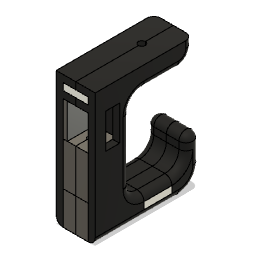
sennheiser_hd280_desk_hanger (Autodesk Fusion 360 design; units mm, degrees)
Autodesk Fusion 360 part; units mm, degrees
note: some values were not read from the file. Set by a fixed rule: which sketch regions a step uses.
sketch "outer_holder" plane through (0, 0, 0) normal (1, 0, 0) x (0, 0, -1)
  line L0 (0, 0) -> (70, 0)
  line L1 (70, 0) -> (70, 0)
  line L2 (60, -10) -> (34.9991, -10)
  line L3 (0, -10) -> (0, 0)
  line L4 (24.9991, -20) -> (24.9991, -65)
  line L5 (24.9991, -90) -> (0, -90)
  line L6 (0, -90) -> (0, -10)
  arc A0 (34.9991, -10) -> (24.9991, -20) centre (34.9991, -20) ccw
  arc A1 (60, -10) -> (70, 0) centre (60, 0) ccw
  line L7 (24.9991, -90) -> (60, -90)
  line L8 (75, -75) -> (75, -75)
  line L9 (55, -75) -> (34.9991, -75)
  line L10 (65, -65) -> (65, -60)
  line L11 (70, -55) -> (70, -55)
  line L12 (75, -60) -> (75, -75)
  arc A2 (70, -55) -> (65, -60) centre (70, -60) ccw
  arc A3 (75, -60) -> (70, -55) centre (70, -60) ccw
  arc A4 (24.9991, -65) -> (34.9991, -75) centre (34.9991, -65) ccw
  arc A5 (55, -75) -> (65, -65) centre (55, -65) ccw
  arc A6 (60, -90) -> (75, -75) centre (60, -75) ccw
  line L13 (7.5, -10) -> (17.5, -10)
  line L14 (17.5, -10) -> (17.5, -35)
  line L15 (17.5, -35) -> (7.5, -35)
  line L16 (7.5, -35) -> (7.5, -10)
  line L17 (35, -85) -> (55, -85)
  line L18 (55, -85) -> (55, -80)
  line L19 (55, -80) -> (35, -80)
  line L20 (35, -80) -> (35, -85)
  line L21 (0, 0) -> (70, 0)
  line L22 (70, 0) -> (70, 5)
  line L23 (70, 5) -> (0, 5)
  line L24 (0, 5) -> (0, 0)
  point P0 (74.9991, -90)
  point P1 (75, -55)
  dimension "d1" = 70
  dimension "d2" = 10
  dimension "d3" = 80
  dimension "d5" = 10
  dimension "d6" = 10
  dimension "d7" = 50
  dimension "d8" = 15
  dimension "d9" = 20
  dimension "d11" = 5
  dimension "d12" = 5
  dimension "d13" = 10
  dimension "d14" = 10
  dimension "d15" = 15
  dimension "d16" = 10
  dimension "d17" = 25
  dimension "d20" = 10
  dimension "d21" = 7.5
  dimension "d55" = 20
  dimension "d56" = 5
  dimension "d122" = 70
  dimension "d123" = 5
  constraint horizontal L0
  constraint horizontal L2
  constraint vertical L3
  constraint coincident L0.start L3.end
  constraint vertical L4
  constraint horizontal L5
  constraint vertical L6
  constraint coincident L3.start L2
  constraint tangent L2 A0
  constraint tangent L4 A0
  constraint tangent L2 A1
  constraint horizontal L7
  constraint horizontal L9
  constraint vertical L10
  constraint vertical L12
  constraint tangent L10 A2
  constraint coincident P1 L12
  constraint coincident P1 L11
  constraint tangent L12 A3
  constraint coincident L5.start L4
  constraint tangent L4 A4
  constraint tangent L9 A4
  constraint coincident L8.start L9
  constraint tangent L10 A5
  constraint tangent L9 A5
  constraint coincident P0 L8
  constraint coincident P0 L7
  constraint tangent L7 A6
  constraint horizontal L13
  constraint vertical L14
  constraint horizontal L15
  constraint vertical L16
  constraint horizontal L17
  constraint vertical L18
  constraint horizontal L19
  constraint vertical L20
  constraint horizontal L21
  constraint vertical L22
  constraint horizontal L23
  constraint vertical L24
  measures "d1" distance of L0.start L0.end
  measures "d2" distance of L0.start L3.start
  measures "d3" distance of L3.start L5.end
  measures "d5" radius of A0
  measures "d6" radius of A1
  measures "d7" distance of L5.start P0
  measures "d8" distance of L7 L9
  measures "d9" distance of L8.start P1
  measures "d11" radius of A2
  measures "d12" radius of A3
  measures "d13" radius of A4
  measures "d14" radius of A5
  measures "d15" radius of A6
  measures "d16" distance of L13.start L13.end
  measures "d17" distance of L13.start L15.end
  measures "d20" distance of L0 L13
  measures "d21" distance of L6 L16
  measures "d55" distance of L17.start L17.end
  measures "d56" distance of L17.start L19.end
  measures "d122" distance of L0.start L0.end
  measures "d123" distance of L0.start L23.end
extrude "Extrude6" add sketch "outer_holder" along normal blind 5 makes body 1
sketch "inner_holder" plane through (5, 0, 0) normal (1, 0, 0) x (0, 0, -1)
  line L0 (15, -35) -> (10, -35)
  line L1 (10, -35) -> (10, -10)
  line L2 (10, -10) -> (15, -10)
  line L3 (15, -10) -> (15, -35)
  line L4 (0, -90) -> (60, -90)
  arc A0 (60, -90) -> (75, -75) centre (60, -75) ccw
  line L5 (75, -75) -> (75, -60)
  arc A1 (75, -60) -> (65, -60) centre (70, -60) ccw
  line L6 (65, -60) -> (65, -65)
  arc A2 (55, -75) -> (65, -65) centre (55, -65) ccw
  line L7 (55, -75) -> (34.9996, -75)
  arc A3 (24.9996, -65) -> (34.9996, -75) centre (34.9996, -65) ccw
  line L8 (24.9996, -65) -> (24.9996, -20)
  arc A4 (34.9996, -10) -> (24.9996, -20) centre (34.9996, -20) ccw
  line L9 (34.9996, -10) -> (60, -10)
  arc A5 (60, -10) -> (70, 0) centre (60, 0) ccw
  line L10 (70, 0) -> (0, 0)
  line L11 (0, 0) -> (0, -55)
  line L12 (0, -55) -> (5, -55)
  line L13 (5, -55) -> (5, -75)
  line L14 (5, -75) -> (0, -75)
  line L15 (0, -75) -> (0, -90)
  line L16 (60, 0) -> (70, 0)
  line L17 (70, 0) -> (70, 0)
  line L18 (0, -10) -> (0, -5)
  arc A6 (60, -10) -> (70, 0) centre (60, 0) ccw
  line L19 (70, -55) -> (70, -55)
  line L20 (65, -60) -> (65, -65)
  line L21 (75, -75) -> (75, -60)
  line L22 (55, -75) -> (35, -75)
  line L23 (20, -90) -> (60, -90)
  line L24 (75, -75) -> (75, -75)
  line L25 (25, -20) -> (25, -65)
  line L26 (20, -90) -> (20, -10)
  arc A7 (35, -10) -> (25, -20) centre (35, -20) ccw
  arc A8 (25, -65) -> (35, -75) centre (35, -65) ccw
  arc A9 (55, -75) -> (65, -65) centre (55, -65) ccw
  arc A10 (70, -55) -> (65, -60) centre (70, -60) ccw
  arc A11 (75, -60) -> (70, -55) centre (70, -60) ccw
  line L27 (0, -10) -> (20, -10)
  arc A12 (60, -90) -> (75, -75) centre (60, -75) ccw
  line L28 (60, 0) -> (60, -10)
  line L29 (35, -10) -> (35, -5)
  line L30 (35, -5) -> (0, -5)
  line L31 (30, -80) -> (60, -80)
  line L32 (60, -80) -> (60, -85)
  line L33 (60, -85) -> (30, -85)
  line L34 (30, -85) -> (30, -80)
  line L35 (17.5, -35) -> (7.5, -35)
  line L36 (7.5, -35) -> (7.5, -10)
  line L37 (7.5, -10) -> (17.5, -10)
  line L38 (17.5, -10) -> (17.5, -35)
  line L39 (35, -85) -> (35, -80)
  line L40 (35, -80) -> (55, -80)
  line L41 (55, -80) -> (55, -85)
  line L42 (55, -85) -> (35, -85)
  line L43 (0, -90) -> (60, -90)
  arc A13 (60, -90) -> (75, -75) centre (60, -75) ccw
  line L44 (75, -75) -> (75, -60)
  arc A14 (75, -60) -> (65, -60) centre (70, -60) ccw
  line L45 (65, -60) -> (65, -65)
  arc A15 (55, -75) -> (65, -65) centre (55, -65) ccw
  line L46 (55, -75) -> (34.9991, -75)
  arc A16 (24.9991, -65) -> (34.9991, -75) centre (34.9991, -65) ccw
  line L47 (24.9991, -65) -> (24.9991, -20)
  arc A17 (34.9991, -10) -> (24.9991, -20) centre (34.9991, -20) ccw
  line L48 (34.9991, -10) -> (60, -10)
  arc A18 (60, -10) -> (70, 0) centre (60, 0) ccw
  line L49 (20, -75) -> (25, -75)
  line L50 (25, -75) -> (25, -85)
  line L51 (25, -85) -> (20, -85)
  line L52 (20, -85) -> (20, -75)
  line L53 (20, -60) -> (25, -60)
  line L54 (25, -60) -> (25, -45)
  line L55 (25, -45) -> (20, -45)
  line L56 (20, -45) -> (20, -60)
  line L57 (70, 0) -> (70, 5)
  line L58 (70, 5) -> (0, 5)
  line L59 (0, 5) -> (0, -90)
  line L60 (60, 0) -> (70, 0)
  line L61 (70, 0) -> (70, 5)
  line L62 (70, 5) -> (60, 5)
  line L63 (60, 5) -> (60, 0)
  dimension "d33" = 10
  dimension "d34" = 10
  dimension "d35" = 10
  dimension "d36" = 10
  dimension "d37" = 5
  dimension "d38" = 5
  dimension "d39" = 15
  dimension "d71" = 5
  dimension "d72" = 10
  dimension "d73" = 5
  dimension "d74" = 15
  dimension "d75" = 5
  dimension "d76" = 35
  dimension "d124" = 10
  dimension "d125" = 5
  constraint horizontal L16
  constraint vertical L18
  constraint vertical L20
  constraint vertical L21
  constraint horizontal L22
  constraint horizontal L23
  constraint coincident L4 L23.start
  constraint vertical L25
  constraint vertical L26
  constraint tangent L25 A7
  constraint tangent L25 A8
  constraint tangent L22 A8
  constraint coincident A0.end L22
  constraint tangent L20 A9
  constraint tangent L22 A9
  constraint tangent L20 A10
  constraint tangent L21 A11
  constraint tangent L23 A12
  constraint coincident A5.centre L16.start
  constraint perpendicular L9 L29
  constraint perpendicular L18 L30
  constraint horizontal L31
  constraint vertical L32
  constraint horizontal L33
  constraint vertical L34
  constraint horizontal L49
  constraint vertical L50
  constraint horizontal L51
  constraint vertical L52
  constraint coincident L26 L49.start
  constraint horizontal L53
  constraint vertical L54
  constraint horizontal L55
  constraint vertical L56
  constraint coincident L26 L53.start
  constraint horizontal L60
  constraint vertical L61
  constraint horizontal L62
  constraint vertical L63
  measures "d33" radius of A6
  measures "d34" radius of A7
  measures "d35" radius of A8
  measures "d36" radius of A9
  measures "d37" radius of A10
  measures "d38" radius of A11
  measures "d39" radius of A12
  measures "d71" distance of L49.start L49.end
  measures "d72" distance of L49.start L51.end
  measures "d73" distance of L23 L51
  measures "d74" distance of L53.start L55.end
  measures "d75" distance of L53.start L53.end
  measures "d76" distance of L9 L55
  measures "d124" distance of A5.centre A5.end
  measures "d125" distance of A5.centre L62.end
extrude "Extrude13" add sketch "inner_holder" along normal blind 9 contours L2 L8 A4 L11 L18 L25 L26 A7 L27 L29 L30 L37 L47 A17 L55 L59 bodies 1
extrude "Extrude14" add sketch "inner_holder" along normal blind 9 contours L4 A0 L5 A1 L6 A2 L7 A3 L8 L20 L21 L22 L23 L25 L26 A8 A9 A10 A11 A12 L43 A13 L44 A14 L45 A15 L46 A16 L47 L49 L50 L51 L53 bodies 1
extrude "Extrude15" add sketch "inner_holder" along normal blind 9 contours L10 L58 L59 L63 | L10 L16 L57 L58 L60 L61 L62 L63 | A5 L10 L16 A6 L28 A18 L60 bodies 1
extrude "Extrude9" add sketch "inner_holder" along normal blind 18 separate body contours L9 L10 L11 L28 L29 L30 L48 L59 makes body 2
extrude "Extrude10" add sketch "outer_holder" along normal blind 5 separate body contours L17 L18 L19 L20 makes body 3
extrude "Extrude11" add sketch "inner_holder" along normal blind 18 contours L31 L33 L34 L39 | L31 L33 L39 L40 L41 L42 | L31 L32 L33 L41 bodies 3
extrude "Extrude12" add sketch "outer_holder" along normal blind 28 contours L17 L18 L19 L20 bodies 3
sketch "plug_side" plane through (5, 0, 0) normal (1, 0, 0) x (0, 0, -1)
  line L0 (20, -90) -> (20, -85)
  line L1 (20, -85) -> (25, -85)
  line L2 (25, -85) -> (25, -75)
  line L3 (25, -75) -> (20, -75)
  line L4 (20, -75) -> (20, -60)
  line L5 (20, -60) -> (24.9991, -60)
  line L6 (24.9991, -60) -> (24.9991, -45)
  line L7 (24.9991, -45) -> (20, -45)
  line L8 (20, -45) -> (20, -10)
  line L9 (20, -10) -> (17.5, -10)
  line L10 (17.5, -10) -> (17.5, -35)
  line L11 (17.5, -35) -> (7.5, -35)
  line L12 (7.5, -35) -> (7.5, -10)
  line L13 (7.5, -10) -> (0, -10)
  line L14 (0, -10) -> (0, -90)
  line L15 (0, -90) -> (20, -90)
  line L16 (0, -66) -> (20, -66)
  line L17 (0, -35) -> (20, -35)
  line L18 (7.5, -10) -> (17.5, -10)
  line L19 (17.5, -10) -> (17.5, -35)
  line L20 (17.5, -35) -> (7.5, -35)
  line L21 (7.5, -35) -> (7.5, -10)
  dimension "d83" = 20
  dimension "d84" = 24
  dimension "d93" = 20
  dimension "d105" = 25
  dimension "d106" = 10
  constraint coincident L14 L16.start
  constraint perpendicular L4 L16
  constraint horizontal L17
  constraint coincident L14 L17.start
  constraint horizontal L18
  constraint vertical L19
  constraint horizontal L20
  constraint vertical L21
  constraint coincident L12.end L13.start
  measures "d83" distance of L16.start L16.end
  measures "d84" distance of L15 L16
  measures "d93" distance of L17.start L17.end
  measures "d105" distance of L12.end L11.end
  measures "d106" distance of L12.end L9.end
extrude "Extrude16" add sketch "plug_side" along normal blind 9 separate body contours L0 L1 L2 L3 L4 L14 L15 L16 makes body 4
sketch "plug_hole_bottom" plane through (0, -90, 0) normal (0, -1, 0) x (1, 0, 0)
  line L0 (5, 0) -> (5, -20)
  line L1 (5, -20) -> (14, -20)
  line L2 (14, -20) -> (14, 0)
  line L3 (14, 0) -> (5, 0)
  arc A0 (14, -4.5) -> (14, -15.5) centre (14, -10) ccw
  arc A1 (14, -6.5) -> (14, -13.5) centre (14, -10) ccw
  dimension "d87" = 5.5
  dimension "d90" = 3.5
  constraint coincident L2 A0.end
  constraint midpoint L2 A0.centre
  constraint coincident L2 A1.end
  constraint coincident L2 A1.start
  constraint coincident A0.centre A1.centre
  measures "d87" radius of A0
  measures "d90" radius of A1
extrude "Extrude17" cut sketch "plug_hole_bottom" against normal blind 22.5 contours L2 A0 A1 | L2 A1 bodies 4
extrude "Extrude18" cut sketch "plug_hole_bottom" against normal blind 24 contours L2 A1 bodies 4
extrude "Extrude19" add sketch "plug_side" along normal blind 9 separate body contours L4 L5 L6 L7 L8 L11 L14 L16 L17 L20 makes body 5
sketch "plug_hole_middle" plane through (0, -66, 0) normal (0, -1, 0) x (1, 0, 0)
  line L0 (5, 0) -> (5, -20)
  line L1 (5, -20) -> (14, -20)
  line L2 (14, -20) -> (14, 0)
  line L3 (14, 0) -> (5, 0)
  arc A0 (14, -5.7) -> (14, -14.3) centre (14, -10) ccw
  arc A1 (14, -7) -> (14, -13) centre (14, -10) ccw
  arc A2 (14, -8.35) -> (14, -11.65) centre (14, -10) ccw
  dimension "d96" = 4.3
  dimension "d97" = 3
  dimension "d102" = 1.65
  constraint coincident L2 A0.end
  constraint midpoint L2 A0.centre
  constraint coincident L2 A1.start
  constraint coincident L2 A1.end
  constraint coincident A0.centre A1.centre
  constraint coincident L2 A2.end
  measures "d96" radius of A0
  measures "d97" radius of A1
  measures "d102" radius of A2
extrude "Extrude20" cut sketch "plug_hole_middle" against normal blind 28 contours L2 A1 A2 | L2 A2 bodies 5
extrude "Extrude21" cut sketch "plug_hole_middle" against normal blind 19 contours L2 A0 A1 bodies 5
extrude "Extrude22" cut sketch "plug_hole_middle" against normal blind 31 contours L2 A2 bodies 5
extrude "Extrude23" add sketch "plug_side" against normal blind 5 separate body contours L10 L11 L12 L17 L18 L19 L20 L21 makes body 6
extrude "Extrude24" add sketch "plug_side" along normal blind 3 contours L10 L11 L12 L17 L18 L19 L20 L21 bodies 6
extrude "Extrude25" add sketch "plug_side" along normal blind 3 contours L12 L13 L14 L17 L21 bodies 6
extrude "Extrude28" add sketch "plug_side" along normal blind 3 contours L8 L9 L10 L17 L19 bodies 6
hole "Hole1" at (14, -10, -47.5) direction (0, 1, 0) diameter 5 depth 15 tip angle 180 countersink diameter 10 countersink angle 90 bodies 2
sketch "screw_hole" plane through (0, 0, 0) normal (0, 1, 0) x (-1, 0, 0)
  circle A0 centre (-14, -47.5) radius 2.5
  line L0 (-5, -60) -> (-5, 0)
  line L1 (-5, 0) -> (-23, 0)
  line L2 (-23, 0) -> (-23, -60)
  line L3 (-23, -60) -> (-5, -60)
  circle A1 centre (-14, -47.5) radius 2.5
  constraint concentric A0 A1
extrude "Extrude27" cut sketch "screw_hole" along normal blind 5 contours A0 A1 bodies 1
fillet "Fillet2" radius 2.5 1 edges at (8.5, -90, -10) on bodies 4
fillet "Fillet3" radius 5 13 edges at (0, 2.5, -70) (0, -7.0711, -67.0711) (0, -10, -47.4996) (0, -12.9289, -27.928) (0, -42.5, -24.9991) (0, -72.0711, -27.928) (0, -75, -44.9996) (0, -72.0711, -62.0711) (0, -62.5, -65) (0, -55, -70) (0, -67.5, -75) (0, -85.6066, -70.6066) (0, -90, -30) on bodies 1
copy_body "CutPasteBodies1" bodies 5 4 1 removing the originals makes body 7 makes body 8 makes body 9 in component "Side"
mirror "MirrorComponent1" about plane through (0, 0, 0) normal (0, 0, 1) of bodies 7 8 9 makes body 10 at (8, -45.3333, 0) makes body 11 at (9.3799, -80.8333, 12.984) makes body 12 at (0, -61.667, 9.1667) in component "Side(Mirror)"
component "Side" placed x (1, 0, 0) y (0, 1, 0) z (0, 0, 1) at (0, 0, 0)
component "Side(Mirror)" placed x (-1, 0, 0) y (0, 1, 0) z (0, 0, -1) at (28, 0, 0)
equation "d69 = 10 mm + 18 mm"
named bodies: "holder_side", "holder_top", "holder_bottom", "plug_bottom", "plug_middle", "plug_top"
